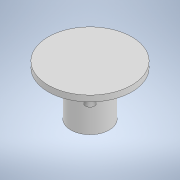
# Autodesk Inventor part: Pieza1
Saved by Autodesk Inventor 2021 (Build 250183000, 183)
## iProperties
Created: 2021-10-13
Part Number: Pieza1
Material: Genérico
Document SubType Name: Modeling
Designer: orgyn
Density: 1 g/cm^3
Appearance: Valor por defecto
Author: orgyn
Autodesk Inventor part; units mm, degrees
ref_plane "YZ Plane" through (0, 0, 0) normal (1, 0, 0) x (0, 1, 0)
ref_plane "XZ Plane" through (0, 0, 0) normal (0, 1, 0) x (-1, 0, 0)
ref_plane "XY Plane" through (0, 0, 0) normal (0, 0, 1) x (1, 0, 0)
sketch "Boceto1" plane through (0, 0, 0) normal (0, 1, 0) x (-1, 0, 0)
  line L0 (0, 0) -> (17, 0)
  line L1 (17, 0) -> (17, -17)
  line L2 (17, -17) -> (0, -17)
  line L3 (0, -17) -> (0, 0)
  circle A0 centre (17, 0) radius 1.5
  circle A1 centre (17, -17) radius 1.5
  circle A2 centre (0, -17) radius 1.5
  circle A3 centre (0, 0) radius 1.5
  circle A4 centre (8.5, -8.5) radius 14.1421
  dimension "d0" = 17
  dimension "d1" = 17
  dimension "d2" = 3
  dimension "d3" = 3
  dimension "d4" = 3
  dimension "d5" = 3
  constraints: 8 end point, 5 centre point, 4 coincident, 3 perpendicular, 1 horizontal
  measures "d0" distance of L0.start L0.end
  measures "d1" distance of L0.end L1.end
  measures "d2" diameter of A0
  measures "d3" diameter of A1
  measures "d4" diameter of A2
  measures "d5" diameter of A3
extrude "Extrusión1" add sketch "Boceto1" along normal blind 2 contours L0 A0 L1 A1 L2 A2 L3 A3 | A4
sketch "Boceto2" plane through (-8.5, 2, -8.5) normal (0, 1, 0) x (1, 0, 0)
  circle A0 centre (8.5, -8.5) radius 1.5
  circle A1 centre (8.5, 8.5) radius 1.5 projected
  circle A2 centre (8.5, 8.5) radius 1.5
  circle A3 centre (-8.5, 8.5) radius 1.5 projected
  circle A4 centre (-8.5, 8.5) radius 1.5
  circle A5 centre (-8.5, -8.5) radius 1.5 projected
  circle A6 centre (-8.5, -8.5) radius 1.5
  constraints: 4 centre point, 4 coincident
extrude "Extrusión2" add sketch "Boceto2" against normal blind 4
sketch "Boceto3" plane through (-8.5, 0, -8.5) normal (0, -1, 0) x (1, 0, 0)
  circle A0 centre (0, 0) radius 6.5
  point P0 (8.5, 8.5)
  dimension "d10" = 13
  constraints: 1 centre point
  measures "d10" diameter of A0
extrude "Extrusión3" add sketch "Boceto3" along normal blind 15
